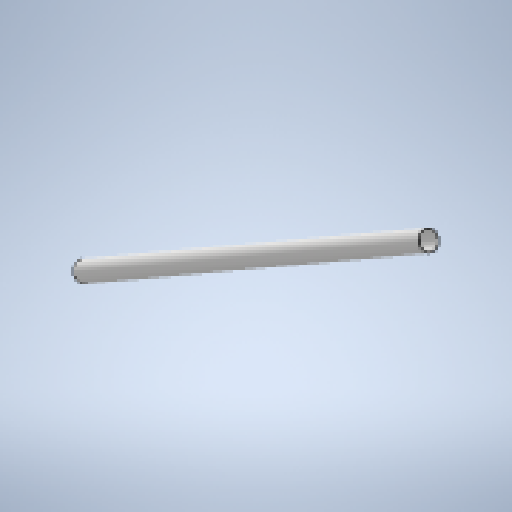
# Autodesk Inventor part: NDM-VOS dummy5
Saved by Autodesk Inventor 2025 (Build 290162010, 162A)
## iProperties
Created: 2024-10-01
Part Number: NDM-VOS dummy5
Material: Generic
Document SubType Name: Modeling
Designer: pokla
Density: 1 g/cm^3
Appearance: Default
Author: pokla
Autodesk Inventor part; units mm, degrees
ref_plane "YZ Plane" through (0, 0, 0) normal (1, 0, 0) x (0, 1, 0)
ref_plane "XZ Plane" through (0, 0, 0) normal (0, 1, 0) x (-1, 0, 0)
ref_plane "XY Plane" through (0, 0, 0) normal (0, 0, 1) x (1, 0, 0)
sketch "Sketch2" plane through (0, 0, 0) normal (0, 1, 0) x (-1, 0, 0)
  line L0 (1503.5082, 1702.7678) -> (-469.8463, 2421.0101)
  line L1 (1503.5082, 1702.7678) -> (-596.4918, 1702.7678) construction
  line L2 (0, 0) -> (0, 2250)
  dimension "d3" = 20
  dimension "d4" = 2100
  dimension "d10" = 2250
  dimension "d11" = 500
  constraints: 6 end point, 1 equal length, 1 horizontal, 1 point on line, 1 vertical
  measures "d3" angle of L1 L0
  measures "d4" distance of L0.start L0.end
  measures "d10" distance of L2.start L2.end
  measures "d11" distance of L0.end L2.end
ref_plane "Work Plane1" through (-1503.5082, 0, 1702.7678) normal (0.9396926, 0, 0.3420201) x (0, 1, 0)
sketch "Sketch3" plane through (-1503.5082, 0, 1702.7678) normal (0.9396926, 0, 0.3420201) x (0, 1, 0)
  circle A0 centre (0, 0) radius 50
  circle A1 centre (0, 0) radius 47
  point P0 (0, -2114.3084)
  point P1 (0, 0)
  point P2 (0, 0)
  point P3 (0, 0)
  dimension "d6" = 100
  dimension "d7" = 3
  constraints: 2 centre point, 1 coincident
  measures "d6" diameter of A0
  measures "d7" radial gap between concentric circles of A0 A1
sweep "Sweep1" add profiles "Sketch3" path "Sketch2" path curves L0
body "Solid2"
